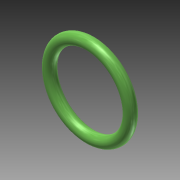
# Autodesk Inventor part: o_ring_4.29_0.5
Saved by Autodesk Inventor 2015 (Build 190159000, 159)
## iProperties
Created: 2015-01-10
Part Number: o_ring_4.29_0.5
Material: Generic
Document SubType Name: Modeling
Designer: ice
Density: 1 g/cm^3
Appearance: Default
Mass: 0.00228235 g
Surface Area: 0.182588 cm^2
Volume: 0.00228235 cm^3
Author: ice
Autodesk Inventor part; units mm, degrees
ref_plane "YZ Plane" through (0, 0, 0) normal (1, 0, 0) x (0, 1, 0)
ref_plane "XY Plane" through (0, 0, 0) normal (0, 0, 1) x (1, 0, 0)
sketch "Sketch1" plane through (0, 0, 0) normal (0, 0, 1) x (1, 0, 0)
  circle A0 centre (1.85, 0) radius 0.25
  line L0 (0, -0.688) -> (0, 1.604)
  line L1 (1.6, 0) -> (0, 0)
  dimension "d3" = 0.5
  dimension "d4" = 1.85
  dimension "d7" = 1.6
  constraints: 4 end point, 1 horizontal, 1 horizontal alignment, 1 vertical, 2 other
  measures "d4" distance of point (1.85, 0) L1.end
  measures "d7" distance of L1.end L1.start
revolve "Revolution1" add sketch "Sketch1" angle 360 about axis through (0, -0.688, 0) along (0, 1, 0)
ref_plane "Work Plane1" through (0, 0.25, 0) normal (0, 1, 0) x (-1, 0, 0)
body "Solid1"
